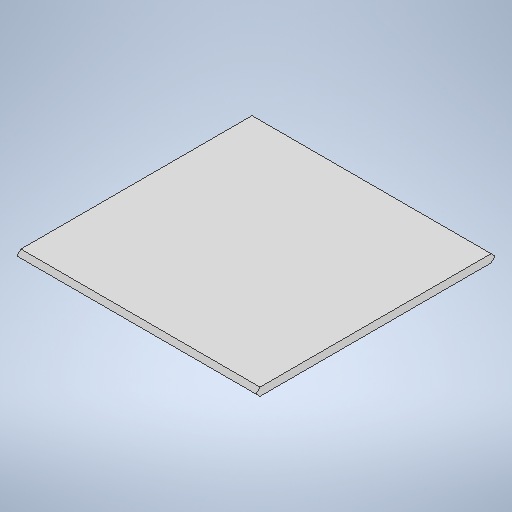
# Autodesk Inventor part: Digital Module Cover V3 Insert
Saved by Autodesk Inventor 2025 (Build 290162000, 162)
## iProperties
Created: 2025-03-18
Part Number: Digital Module Cover V3 Insert
Material: Generic
Document SubType Name: Modeling
Designer: Caleb Fangmeier
Density: 1 g/cm^3
Appearance: Default
Author: Caleb Fangmeier
Autodesk Inventor part; units mm, degrees
ref_plane "YZ Plane" through (0, 0, 0) normal (1, 0, 0) x (0, 1, 0)
ref_plane "XZ Plane" through (0, 0, 0) normal (0, 1, 0) x (-1, 0, 0)
ref_plane "XY Plane" through (0, 0, 0) normal (0, 0, 1) x (1, 0, 0)
sketch "Sketch1" plane through (0, 0, 0) normal (0, 1, 0) x (-1, 0, 0)
  line L0 (-22.4, -22.4) -> (22.4, -22.4)
  line L1 (22.4, -22.4) -> (22.4, 22.4)
  line L2 (22.4, 22.4) -> (-22.4, 22.4)
  line L3 (-22.4, 22.4) -> (-22.4, -22.4)
  line L4 (-22.4, -22.4) -> (22.4, 22.4) construction
  line L5 (22.4, -22.4) -> (-22.4, 22.4) construction
  point P0 (0, 0)
  dimension "d0" = 44.8
  dimension "d1" = 44.8
  constraints: 12 end point, 2 midpoint, 2 parallel, 1 horizontal, 1 perpendicular
  measures "d0" distance of L0.end L1.end
  measures "d1" distance of L1.end L2.end
extrude "Extrusion1" add sketch "Sketch1" along normal blind 1.5
sketch "Sketch2" plane through (22.4, 0, 22.4) normal (1, 0, 0) x (0, 0, -1)
  line L0 (44.8, 0) -> (0, 0) projected
  line L1 (0.75, 1.5) -> (0, 0.75)
  line L2 (0.75, 1.5) -> (1.8107, 1.5) construction
  line L3 (0, 0.75) -> (0.75, 0)
  line L4 (0, 0) -> (0, 1.5) projected
  line L5 (22.4, -4.0308) -> (22.4, 6.4537)
  line L6 (0.75, 1.5) -> (0, 1.5)
  line L7 (0, 1.5) -> (0, 0)
  line L8 (0.75, 0) -> (0, 0)
  line L9 (0, 1.5) -> (44.8, 1.5) projected
  line L10 (0, 0) -> (44.8, 0)
  line L11 (44.05, 1.5) -> (44.8, 0.75)
  line L12 (44.05, 1.5) -> (42.9893, 1.5) construction
  line L13 (44.8, 0.75) -> (44.05, 0)
  line L14 (44.8, 0) -> (44.8, 1.5)
  line L15 (44.05, 1.5) -> (44.8, 1.5)
  line L16 (44.8, 1.5) -> (44.8, 0)
  line L17 (44.05, 0) -> (44.8, 0)
  line L18 (44.8, 1.5) -> (0, 1.5)
  point P0 (22.4, 0)
  point P1 (22.4, 0)
  dimension "d7" = 45
  dimension "d8" = 45
  constraints: 32 end point, 8 symmetric about line, 5 point on line, 3 midpoint, 2 collinear, 1 equal length, 1 horizontal, 1 vertical, 1 vertical alignment
  measures "d7" angle of L4 L1
  measures "d8" angle of L4 L3
extrude "Extrusion2" cut sketch "Sketch2" against normal through all contours L0 L13 L14 | L11 L9 L14 | L0 L4 L3 | L4 L6 L1
body "Solid1"
